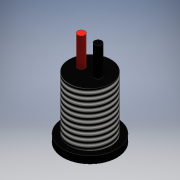
# Autodesk Inventor part: USB plug
Saved by Autodesk Inventor 2016 (Build 200138000, 138)
## iProperties
Created: 2019-09-20
Part Number: USB plug
Material: Generic
Document SubType Name: Modeling
Designer: jimmy
Density: 1 g/cm^3
Appearance: Default
Author: jimmy
Autodesk Inventor part; units mm, degrees
ref_plane "YZ Plane" through (0, 0, 0) normal (1, 0, 0) x (0, 1, 0)
ref_plane "XZ Plane" through (0, 0, 0) normal (0, 1, 0) x (-1, 0, 0)
ref_plane "XY Plane" through (0, 0, 0) normal (0, 0, 1) x (1, 0, 0)
sketch "Sketch1" plane through (0, 0, 0) normal (0, 0, 1) x (1, 0, 0)
  circle A0 centre (0, 0) radius 14.39
  dimension "d0" = 28.78
  constraints: 1 centre point, 1 coincident
  measures "d0" diameter of A0
extrude "Extrusion1" add sketch "Sketch1" along normal blind 37
sketch "Sketch2" plane through (0, 0, 37) normal (0, 0, 1) x (1, 0, 0)
  circle A0 centre (-5.9617, 0) radius 2.5
  circle A1 centre (5.5337, 0) radius 2.5
  point P0 (0, 0)
  dimension "d3" = 5
  dimension "d4" = 5
  constraints: 2 centre point
  measures "d3" diameter of A0
  measures "d4" diameter of A1
extrude "Extrusion2" add sketch "Sketch2" along normal blind 20
sketch "Sketch3" plane through (0, 0, 0) normal (0, 0, -1) x (-1, 0, 0)
  circle A0 centre (0, 0) radius 18.5
  dimension "d7" = 37
  constraints: 1 centre point, 1 coincident
  measures "d7" diameter of A0
extrude "Extrusion3" add sketch "Sketch3" along normal blind 5
sketch "Sketch4" plane through (0, 0, -5) normal (0, 0, -1) x (-1, 0, 0)
  line L0 (-6.8621, 5.2759) -> (7.1379, 5.2759)
  line L1 (7.1379, 5.2759) -> (7.1379, 9.2759)
  line L2 (7.1379, 9.2759) -> (-6.8621, 9.2759)
  line L3 (-6.8621, 9.2759) -> (-6.8621, 5.2759)
  line L4 (-6.8621, 5.2759) -> (7.1379, 9.2759) construction
  line L5 (7.1379, 5.2759) -> (-6.8621, 9.2759) construction
  line L6 (-6.8621, -9.069) -> (7.1379, -9.069)
  line L7 (7.1379, -9.069) -> (7.1379, -5.069)
  line L8 (7.1379, -5.069) -> (-6.8621, -5.069)
  line L9 (-6.8621, -5.069) -> (-6.8621, -9.069)
  line L10 (-6.8621, -9.069) -> (7.1379, -5.069) construction
  line L11 (7.1379, -9.069) -> (-6.8621, -5.069) construction
  point P0 (0, 0)
  point P1 (0.1379, 7.2759)
  point P2 (0.1379, -7.069)
  dimension "d10" = 4
  dimension "d11" = 14
  dimension "d12" = 14
  dimension "d13" = 4
  constraints: 24 end point, 4 midpoint, 4 parallel, 2 horizontal, 2 perpendicular, 1 point on line
  measures "d10" distance of L0.end L1.end
  measures "d11" distance of L1.end L2.end
  measures "d12" distance of L7.end L8.end
  measures "d13" distance of L6.end L7.end
extrude "Extrusion4" cut sketch "Sketch4" against normal blind 2
thread "Thread1" size "M30x3.5" class "6g" standard "ANSI Metric M Profile" full length
equation "\"d12\" = d11"
equation "\"d13\" = d10"
body "Solid1"
